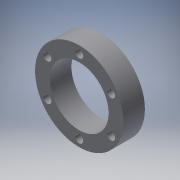
# Autodesk Inventor part: spacer
Saved by Autodesk Inventor 2016 (Build 200138000, 138)
## iProperties
Created: 2016-01-17
Part Number: spacer
Material: Generic
Document SubType Name: Modeling
Designer: gus
Mass: 18.1413 g
Surface Area: 81.4198 cm^2
Volume: 18.1413 cm^3
Density: 1 g/cm^3
Appearance: Default
Author: gus
Autodesk Inventor part; units mm, degrees
ref_plane "YZ Plane" through (0, 0, 0) normal (1, 0, 0) x (0, 1, 0)
ref_plane "XZ Plane" through (0, 0, 0) normal (0, 1, 0) x (-1, 0, 0)
ref_plane "XY Plane" through (0, 0, 0) normal (0, 0, 1) x (1, 0, 0)
sketch "Sketch1" plane through (0, 0, 0) normal (0, 0, 1) x (1, 0, 0)
  circle A0 centre (0, 0) radius 28.575
  circle A1 centre (0, 0) radius 23.8125 construction
  line L0 (0, 23.8125) -> (20.6222, 11.9063) construction
  line L1 (20.6222, 11.9063) -> (20.6222, -11.9063) construction
  line L2 (20.6222, -11.9063) -> (0, -23.8125) construction
  line L3 (0, -23.8125) -> (-20.6222, -11.9062) construction
  line L4 (-20.6222, -11.9062) -> (-20.6222, 11.9063) construction
  line L5 (-20.6222, 11.9063) -> (0, 23.8125) construction
  circle A2 centre (0, 23.8125) radius 2.5908
  circle A3 centre (-20.6222, 11.9063) radius 2.5908
  circle A4 centre (-20.6222, -11.9062) radius 2.5908
  circle A5 centre (0, -23.8125) radius 2.5908
  circle A6 centre (20.6222, -11.9063) radius 2.5908
  circle A7 centre (20.6222, 11.9063) radius 2.5908
  circle A8 centre (0, 0) radius 19.05
  dimension "d0" = 57.15
  dimension "d1" = 47.625
  dimension "d2" = 5.1816
  dimension "d3" = 5.1816
  dimension "d4" = 5.1816
  dimension "d5" = 5.1816
  dimension "d6" = 5.1816
  dimension "d7" = 5.1816
  dimension "d8" = 38.1
  constraints: 12 end point, 9 centre point, 9 coincident, 2 point on circle, 1 point on line, 1 vertical, 13 other
  measures "d0" diameter of A0
  measures "d1" diameter of A1
  measures "d2" diameter of A2
  measures "d3" diameter of A3
  measures "d4" diameter of A4
  measures "d5" diameter of A5
  measures "d6" diameter of A6
  measures "d7" diameter of A7
  measures "d8" diameter of A8
extrude "Extrusion1" add sketch "Sketch1" against normal blind 13.97
body "Solid1"
